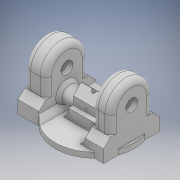
# Autodesk Inventor part: BasePan
Saved by Autodesk Inventor 2017 (Build 210142000, 142)
## iProperties
Created: 2016-12-30
Part Number: BasePan
Material: Generic
Document SubType Name: Modeling
Designer: Samanth
Density: 1 g/cm^3
Appearance: Default
Author: Samanth
Autodesk Inventor part; units mm, degrees
ref_plane "YZ Plane" through (0, 0, 0) normal (1, 0, 0) x (0, 1, 0)
ref_plane "XZ Plane" through (0, 0, 0) normal (0, 1, 0) x (-1, 0, 0)
ref_plane "XY Plane" through (0, 0, 0) normal (0, 0, 1) x (1, 0, 0)
sketch "Sketch1" plane through (0, 0, 0) normal (0, 0, 1) x (1, 0, 0)
  circle A0 centre (0, 0) radius 75
  dimension "d0" = 150
  constraints: 1 centre point, 1 coincident
  measures "d0" diameter of A0
extrude "Extrusion1" add sketch "Sketch1" along normal blind 10
sketch "Sketch2" plane through (0, 0, 10) normal (0, 0, 1) x (1, 0, 0)
  circle A0 centre (0, 0) radius 4.4
  dimension "d3" = 8.8
  constraints: 1 centre point, 1 coincident
  measures "d3" diameter of A0
extrude "Extrusion2" cut sketch "Sketch2" against normal blind 10
sketch "Sketch3" plane through (0, 0, 10) normal (0, 0, 1) x (1, 0, 0)
  circle A0 centre (0, 0) radius 75 projected
  line L0 (-52.6833, -53.3804) -> (52.6833, -53.3804)
  line L1 (52.6833, -53.3804) -> (52.6833, 53.3804)
  line L2 (52.6833, 53.3804) -> (-52.6833, 53.3804)
  line L3 (-52.6833, 53.3804) -> (-52.6833, -53.3804)
  line L4 (-52.6833, -53.3804) -> (52.6833, 53.3804) construction
  line L5 (52.6833, -53.3804) -> (-52.6833, 53.3804) construction
  line L6 (-52.6833, 53.3804) -> (-92.6833, 53.3804)
  line L7 (-92.6833, 53.3804) -> (-92.6833, -53.3804)
  line L8 (-92.6833, -53.3804) -> (-52.6833, -53.3804)
  line L9 (-52.6833, -53.3804) -> (-52.6833, 53.3804)
  line L10 (35.6171, 53.3804) -> (70.6171, 53.3804)
  line L11 (70.6171, 53.3804) -> (70.6171, -53.3804)
  line L12 (70.6171, -53.3804) -> (35.6171, -53.3804)
  line L13 (35.6171, -53.3804) -> (35.6171, 53.3804)
  dimension "d6" = 40
  dimension "d7" = 35
  constraints: 28 end point, 6 parallel, 3 horizontal, 3 perpendicular, 2 midpoint, 2 point on line, 2 other
  measures "d6" distance of L8.end L7.end
  measures "d7" distance of L11.end L12.end
extrude "Extrusion3" add sketch "Sketch3" along normal blind 60 and the other way blind 10 contours L10 L11 A0 | A0 L11 L1 | L1 L0 L13 L2 | L3 A0 | A0 L8 L7 L6 | A0 L11 L12
sketch "Sketch4" plane through (70.6171, -25.2631, 10) normal (1, 0, 0) x (0, 0, -1)
  line L0 (-60, 78.6435) -> (-60, -28.1174) projected
  circle A0 centre (-60, 25.2631) radius 4.4
  point P0 (10, 25.2631)
  dimension "d12" = 8.8
  constraints: 1 centre point, 1 midpoint
  measures "d12" diameter of A0
extrude "Extrusion4" cut sketch "Sketch4" against normal blind 1660
sketch "Sketch5" plane through (70.6171, -25.2631, 10) normal (1, 0, 0) x (0, 0, -1)
  arc A0 (-60, 20.8631) -> (-60, 29.6631) centre (-60, 25.2631) ccw projected
  circle A1 centre (-60, 25.2631) radius 40
  point P0 (10, 25.2631)
  dimension "d15" = 80
  constraints: 1 centre point, 1 coincident
  measures "d15" diameter of A1
extrude "Extrusion5" add sketch "Sketch5" against normal up to surface (35 mm away)
sketch "Sketch6" plane through (-92.6833, -53.3804, 0) normal (-1, 0, 0) x (0, 0, 1)
  arc A0 (70, 57.7804) -> (70, 48.9804) centre (70, 53.3804) ccw projected
  circle A1 centre (70, 53.3804) radius 40
  point P0 (0, 53.3804)
  constraints: 1 centre point, 1 coincident
extrude "Extrusion6" add sketch "Sketch6" against normal up to surface (40 mm away)
sketch "Sketch7" plane through (-92.6833, -53.3804, 0) normal (-1, 0, 0) x (0, 0, 1)
  circle A0 centre (70, 53.3804) radius 11.5
  point P0 (0, 53.3804)
  dimension "d20" = 23
  constraints: 1 centre point
  measures "d20" diameter of A0
extrude "Extrusion7" cut sketch "Sketch7" against normal blind 10
sketch "Sketch8" plane through (-52.6833, -53.3804, 10) normal (1, 0, 0) x (0, 0, -1)
  circle A0 centre (-60, 53.3804) radius 11.5 projected
  circle A1 centre (-60, 53.3804) radius 11.5
  point P0 (10, 53.3804)
  constraints: 1 centre point, 1 coincident
extrude "Extrusion8" cut sketch "Sketch8" against normal blind 10 and the other way blind 99.25
sketch "Sketch9" plane through (70.6171, -25.2631, 10) normal (1, 0, 0) x (0, 0, -1)
  circle A0 centre (-60, 25.2631) radius 11.5 projected
  circle A1 centre (-60, 25.2631) radius 11.5
  point P0 (10, 25.2631)
  constraints: 1 centre point, 1 coincident
extrude "Extrusion9" cut sketch "Sketch9" against normal blind 10
sketch "Sketch10" plane through (60.6171, 0, 70) normal (1, 0, 0) x (0, 0, -1)
  circle A0 centre (0, 0) radius 11.5 projected
  circle A1 centre (0, 0) radius 5.0409
  point P0 (70, 0)
  constraints: 1 centre point, 1 coincident
extrude "Extrusion10" cut sketch "Sketch10" against normal blind 200 contours A1
sketch "Sketch11" plane through (0, 0, 10) normal (0, 0, 1) x (1, 0, 0)
  line L0 (-25.0777, -24.5658) -> (25.0777, -24.5658)
  line L1 (25.0777, -24.5658) -> (25.0777, 24.5658)
  line L2 (25.0777, 24.5658) -> (-25.0777, 24.5658)
  line L3 (-25.0777, 24.5658) -> (-25.0777, -24.5658)
  line L4 (-25.0777, -24.5658) -> (25.0777, 24.5658) construction
  line L5 (25.0777, -24.5658) -> (-25.0777, 24.5658) construction
  point P0 (0, 0)
  constraints: 12 end point, 2 midpoint, 2 parallel, 1 horizontal, 1 perpendicular
extrude "Extrusion11" add sketch "Sketch11" along normal blind 50
sketch "Sketch12" plane through (-25.0777, -24.5658, 10) normal (0, -1, 0) x (1, 0, 0)
  circle A0 centre (25.0777, 25) radius 2.5
  point P0 (25.0777, -10)
  dimension "d33" = 5
  constraints: 1 centre point
  measures "d33" diameter of A0
extrude "Extrusion12" cut sketch "Sketch12" against normal blind 59.25
sketch "Sketch13" plane through (0, 0, 10) normal (0, 0, -1) x (-1, 0, 0)
  circle A0 centre (0, 0) radius 4.3737
  constraints: 1 centre point, 1 coincident
extrude "Extrusion13" cut sketch "Sketch13" against normal blind 51.25
sketch "Sketch14" plane through (0, 0, 60) normal (0, 0, 1) x (1, 0, 0)
  line L0 (25.0777, 24.5658) -> (25.0777, -24.5658) projected
  line L1 (-25.0777, 15.3587) -> (25.0777, 15.3587)
  line L2 (25.0777, 15.3587) -> (25.0777, -15.3587)
  line L3 (25.0777, -15.3587) -> (-25.0777, -15.3587)
  line L4 (-25.0777, -15.3587) -> (-25.0777, 15.3587)
  circle A0 centre (0, 0) radius 4.3737 projected
  line L5 (-25.0777, 15.3587) -> (25.0777, -15.3587) construction
  line L6 (25.0777, 15.3587) -> (-25.0777, -15.3587) construction
  line L7 (-25.0777, 24.5658) -> (25.0777, 24.5658) projected
  line L8 (25.0777, 15.3587) -> (-25.0777, 15.3587)
  line L9 (-25.0777, 15.3587) -> (-25.0777, 24.5658)
  line L10 (-25.0777, 24.5658) -> (25.0777, 24.5658)
  line L11 (25.0777, 24.5658) -> (25.0777, 15.3587)
  line L12 (25.0777, -24.5658) -> (-25.0777, -24.5658) projected
  line L13 (-25.0777, -15.3587) -> (25.0777, -15.3587)
  line L14 (25.0777, -15.3587) -> (25.0777, -24.5658)
  line L15 (25.0777, -24.5658) -> (-25.0777, -24.5658)
  line L16 (-25.0777, -24.5658) -> (-25.0777, -15.3587)
  constraints: 28 end point, 6 parallel, 3 horizontal, 3 perpendicular, 2 midpoint, 1 point on line
extrude "Extrusion14" cut sketch "Sketch14" against normal blind 30.25 contours L0 L1 L9 L7 | L0 L12 L16 L3
chamfer "Chamfer3" distance 15 angle 45 2 edges at (0, 15.3587, 60) (0, -15.3587, 60)
chamfer "Chamfer4" distance 10 angle 45 4 edges at (25.0777, 0, 10) (-25.0777, 0, 10) (35.6171, 0, 10) (-52.6833, 0, 10)
sketch "Sketch15" plane through (-25.0777, -24.5658, 29.75) normal (-1, 0, 0) x (0, 0, 1)
  line L0 (0, 0) -> (0, 9.2071) projected
  circle A0 centre (0, 24.5658) radius 15.3587
  point P0 (-29.75, 24.5658)
  constraints: 1 vertical alignment, 2 other
extrude "Extrusion15" add sketch "Sketch15" along normal blind 30.25 and the other way blind 61.875
sketch "Sketch16" plane through (0, 0, 0) normal (0, 0, -1) x (-1, 0, 0)
  circle A0 centre (0, 0) radius 4.4
  constraints: 1 centre point, 1 coincident
extrude "Extrusion16" cut sketch "Sketch16" against normal blind 58.75
sketch "Sketch17" plane through (-25.0777, 15.3587, 45) normal (0, 1, 0) x (1, 0, 0)
  circle A0 centre (25.0777, 10) radius 2.5 projected
  circle A1 centre (25.0777, 10) radius 2.5
  point P0 (25.0777, 45)
  constraints: 1 centre point, 1 coincident
extrude "Extrusion17" cut sketch "Sketch17" against normal blind 58.75
chamfer "Chamfer5" distance 6 angle 45 3 edges at (-52.6833, -13.8859, 36.3129) (-52.6833, 13.8859, 36.3129) (35.6171, 0, 45.1087)
sketch "Sketch18" plane through (0, 0, 70) normal (0, 0, 1) x (1, 0, 0)
  line L0 (-52.6833, -53.3804) -> (-92.6833, -53.3804) projected
  line L1 (70.6171, -53.3804) -> (70.6171, -40) projected
  line L2 (-92.6833, -53.3804) -> (70.6171, -53.3804)
  line L3 (70.6171, -53.3804) -> (70.6171, -40)
  line L4 (70.6171, -40) -> (-92.6833, -40)
  line L5 (-92.6833, -40) -> (-92.6833, -53.3804)
  line L6 (-92.6833, 40) -> (-52.6833, 40) projected
  line L7 (70.6171, 53.3804) -> (70.6171, 25.2631) projected
  line L8 (-92.6833, 40) -> (70.6171, 40)
  line L9 (70.6171, 40) -> (70.6171, 53.3804)
  line L10 (70.6171, 53.3804) -> (-92.6833, 53.3804)
  line L11 (-92.6833, 53.3804) -> (-92.6833, 40)
  point P0 (0, 0)
  constraints: 16 end point, 4 parallel, 2 horizontal, 2 perpendicular
extrude "Extrusion18" cut sketch "Sketch18" against normal blind 32.75
chamfer "Chamfer7" distance 13 angle 45 4 edges at (-72.6833, -53.3804, 37.25) (53.1171, -53.3804, 37.25) (-72.6833, 53.3804, 37.25) (53.1171, 53.3804, 37.25)
fillet "Fillet3" radius 11 12 edges at (-92.6833, -40, 53.625) (-92.6833, 40, 53.625) (-92.6833, 0, 110) (-52.6833, 40, 53.625) (-52.6833, -40, 53.625) (-52.6833, 0, 110) (35.6171, -40, 53.625) (35.6171, 40, 53.625) (35.6171, 0, 110) (70.6171, 40, 53.625) (70.6171, -40, 53.625) (70.6171, 0, 110)
body "Solid1"
